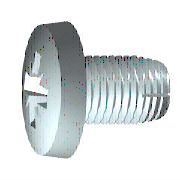
# Autodesk Inventor part: ANSI B18.6.5M - M3x0.5 x 16
Saved by Autodesk Inventor 2013 (Build 170138000, 138)
## iProperties
Created: 2012-02-10
Part Number: ANSI B18.6.5M - M3x0.5 x 16
Material: Steel, Mild
Description: Cross Recessed Pan Head Tapping Screw - Type D - Type IA - Metric
Document SubType Name: Modeling
Standard: ANSI B18.6.5M
Designer: Nico
Standard Revision: 2000
Standards Organization: ANSI
Language: en-US
Size Designation: M3x0.5 x 16
Categories: <MemberInstance><Categories><Category DisplayName="Fasteners" InternalName="e4da775c-781d-43d5-af7c-5136215cf5a6" Mnemonic="FSTN"><Category DisplayName="Bolts" InternalName="536e6df0-f778-49ac-b2f2-25c71d2aa0b2" Mnemonic="SCRW"><CategoryParameter DisplayName="Nominal Diameter" InternalName="8bbe3f8e-44cf-40a9-a251-3a6edc8168d6" Mnemonic="nomdia"/><CategoryParameter DisplayName="Nominal Length" InternalName="238ecbaf-3e6c-45dd-aa95-4068c8e0fd02" Mnemonic="nomlen"/><CategoryParameter DisplayName="Thread Series Designation" InternalName="87c5849c-b3a5-4c3e-9c9b-2feecef9be86" Mnemonic="thrserdsgn"/><CategoryParameter DisplayName="Thread Class" InternalName="ebc0d23b-2cc6-4d2a-b376-d52aae53bab6" Mnemonic="thrclss"/><CategoryParameter DisplayName="Thread Designation" InternalName="586d5e89-370a-4089-914f-0110033585c7" Mnemonic="thrdesign"/><CategoryParameter DisplayName="Thread Type" InternalName="b4bbb7bc-d6aa-4c9f-a9a9-4152b9f6fe49" Mnemonic="thrtype"/><CategoryParameter DisplayName="Threads per Unit" InternalName="bdc6e7d2-ffd0-4d9c-a173-16b95ebb912d" Mnemonic="thrperunit1"/><CategoryParameter DisplayName="Thread Pitch" InternalName="bb82302e-82d8-4176-8fc1-c5d7bb17d5ad" Mnemonic="pitch1"/><CategoryParameter DisplayName="Nominal Diameter Designation" InternalName="03caf894-eafd-4c09-a035-916ac084b87b" Mnemonic="nomdiadesig"/><Category DisplayName="Round Head" InternalName="df3578aa-538f-4805-96a8-2439eb0c3cf7" Mnemonic="RNDSCRW"><CategoryParameter DisplayName="Shank Diameter" InternalName="c22f1a48-b8d5-43ef-ac5e-546ba91c0bd6" Mnemonic="grpdia"/><CategoryParameter DisplayName="Grip Length" InternalName="2c6ace26-543b-4217-91c4-9cdf8c3ec6f1" Mnemonic="grplen"/><CategoryParameter DisplayName="Thread Length" InternalName="a1e5edc5-4ca7-4847-8786-65b14d35af16" Mnemonic="thrlen"/><CategoryParameter DisplayName="Head Diameter" InternalName="e71ee7a1-06fd-425c-ba3b-09769885677c" Mnemonic="headdia"/><CategoryParameter DisplayName="Head Height" InternalName="2d152238-84fe-49ae-94c3-3fee884c292b" Mnemonic="headh"/><CategoryParameter DisplayName="Property Class" InternalName="85496db6-1567-48ed-b0d4-aa1f03366005" Mnemonic="propclss"/><Category DisplayName="Self Tapping Screws" InternalName="33fb404f-0d7c-4133-a804-5105a5fcc9da" Mnemonic="RNDCNRGTPSCRW"/></Category></Category></Category><Category DisplayName="DataType" InternalName="23b78d0f-2648-40c6-8793-ca6db495c9e8" Mnemonic="DATATYPE"><CategoryParameter DisplayName="DisplayName" InternalName="05415f3d-3907-474b-a020-eb9d644f4cf3" Mnemonic="DISPLAYNAME"/><CategoryParameter DisplayName="InternalName" InternalName="cf1d0246-76d9-4b4a-8305-fa0409afb5c1" Mnemonic="INTERNALNAME"/><CategoryParameter DisplayName="Folder Name" InternalName="3f06958e-8713-4116-9be7-ed6184ecc97b" Mnemonic="FOLDERNAME"/><CategoryParameter DisplayName="Family Version" InternalName="914462f6-6e19-4b14-ba84-155b9680b1d0" Mnemonic="FAMILYREVISION"/><CategoryParameter DisplayName="ClipFormat" InternalName="bc51e27b-3422-4e78-93ef-cec197ddf230" Mnemonic="CLIPFORMAT"/><CategoryParameter DisplayName="IsMetric" InternalName="e2385c5b-1ea4-4823-96a8-8de651266ec3" Mnemonic="ISMETRIC"/><CategoryParameter DisplayName="Description" InternalName="13903e3d-64b1-4950-80da-f627842ea37f" Mnemonic="DESCRIPTION"/><CategoryParameter DisplayName="StdsOrg" InternalName="8f5914e1-4693-403f-8ab5-d37768198c9d" Mnemonic="STDSORG"/><CategoryParameter DisplayName="Standard" InternalName="0c0a119c-1e12-4c84-803f-101930972f5e" Mnemonic="STANDARD"/><CategoryParameter DisplayName="Manufacturer" InternalName="cd6c7a72-a28a-4e50-99a9-2c7f4e13e5ad" Mnemonic="MANUFACTURER"/><CategoryParameter DisplayName="Member Revision" InternalName="a65d44b9-392f-4f4f-857b-e4b3d54996fe" Mnemonic="MEMBERREVISION"/><CategoryParameter DisplayName="Standard Revision" InternalName="91d5a463-65c2-4fde-b823-3b7fea5e8e17" Mnemonic="STANDARDREVISION"/><CategoryParameter DisplayName="Revision Guid" InternalName="45a75005-10b1-4dfc-8d6d-dfe629f0b93c" Mnemonic="REVISIONGUID"/><CategoryParameter DisplayName="Designation" InternalName="2675968c-4ce5-49e0-a4f5-552d29089031" Mnemonic="DESIGNATION"/><CategoryParameter DisplayName="FileName" InternalName="8b46a4cc-9585-4fed-90c3-899f57e09a73" Mnemonic="FILENAME"/><CategoryParameter DisplayName="Default Row" InternalName="2af9ec52-faaa-4026-b378-f9fa4afca842" Mnemonic="DEFAULTROW"/><Category DisplayName="Part" InternalName="c0e0b642-3bcb-4cc8-9e80-f96d35c4afa4" Mnemonic="PART"><CategoryParameter DisplayName="Material" InternalName="818a152a-d3c3-49ca-80ee-df7d91421b8e" Mnemonic="MATERIAL"/><CategoryParameter DisplayName="Material Key" InternalName="5c9a8adb-dd2b-4535-b97f-0a94a95fe41f" Mnemonic="MATERIALKEY"/><CategoryParameter DisplayName="Part Number" InternalName="016b6077-bfbe-49bd-92c9-d8d59c39c941" Mnemonic="PARTNUMBER"/><CategoryParameter DisplayName="Stock Number" InternalName="4dba7c1c-e26c-444e-836c-b08b433409a8" Mnemonic="STOCKNUMBER"/></Category></Category><Category DisplayName="LegacyMap" InternalName="cd87c42b-3e48-431e-b5c0-1cbeb14dfe77" Mnemonic="LEGACYMAP"><CategoryParameter DisplayName="CatalogName" InternalName="d99d1e27-aa94-4de2-af4c-c348882a6f4f" Mnemonic="CATALOGNAME"/><CategoryParameter DisplayName="FamilyNumber" InternalName="e705e1f4-09cb-413e-91f9-551b4188271e" Mnemonic="FAMILYNUMBER"/><CategoryParameter DisplayName="MemberID" InternalName="8e5e0294-fc51-4c8f-b3d7-003dc5ed94f6" Mnemonic="MEMBERID"/><CategoryParameter DisplayName="unique CC member ID" InternalName="5193edd4-b2b0-4ab4-9d54-de900eee34e0" Mnemonic="CCCOOKIE"/><CategoryParameter DisplayName="unique DA member ID" InternalName="0918ad47-427f-4fed-ae26-24c81c58f590" Mnemonic="DACOOKIE"/><CategoryParameter DisplayName="Merge11 ID" InternalName="0ee8fb18-e2ed-4f39-96f6-1f4b5f50aa71" Mnemonic="MERGE11"/><CategoryParameter DisplayName="Split ID" InternalName="72b5c83c-be7f-45c4-ae51-9160ea6deb26" Mnemonic="SPLIT"/></Category></Categories><FamilyTemplate Id="si1048"><FamilyTemplateParameters><FamilyTemplateParameter ObjectType="kUserParameterObject" ValueType="xs:double" Id="1" ObjectReferenceKey="GUL"/><FamilyTemplateParameter ObjectType="kUserParameterObject" ValueType="xs:double" Id="2" ObjectReferenceKey="KOH"/><FamilyTemplateParameter ObjectType="kUserParameterObject" ValueType="xs:double" Id="3" ObjectReferenceKey="GD2"/><FamilyTemplateParameter ObjectType="kUserParameterObject" ValueType="xs:double" Id="4" ObjectReferenceKey="KOD"/><FamilyTemplateParameter ObjectType="kUserParameterObject" ValueType="xs:double" Id="5" ObjectReferenceKey="SBR"/><FamilyTemplateParameter ObjectType="kUserParameterObject" ValueType="xs:double" Id="6" ObjectReferenceKey="KR"/><FamilyTemplateParameter ObjectType="kUserParameterObject" ValueType="xs:double" Id="7" ObjectReferenceKey="GEL"/><FamilyTemplateParameter ObjectType="kUserParameterObject" ValueType="xs:double" Id="8" ObjectReferenceKey="THREADDIA"/><FamilyTemplateParameter ObjectType="kUserParameterObject" ValueType="xs:double" Id="9" ObjectReferenceKey="TOA"/><FamilyTemplateParameter ObjectType="kUserParameterObject" ValueType="xs:double" Id="10" ObjectReferenceKey="NLG"/><FamilyTemplateParameter ObjectType="kUserParameterObject" ValueType="xs:double" Id="11" ObjectReferenceKey="STI"/><FamilyTemplateParameter ObjectType="kUserParameterObject" ValueType="xs:double" Id="12" ObjectReferenceKey="TPU"/><FamilyTemplateParameter ObjectType="kUserParameterObject" ValueType="xs:double" Id="13" ObjectReferenceKey="PTC"/><FamilyTemplateParameter ObjectType="kUserParameterObject" ValueType="xs:double" Id="14" ObjectReferenceKey="SDM"/><FamilyTemplateParameter ObjectType="kUserParameterObject" ValueType="xs:double" Id="15" ObjectReferenceKey="NND"/><FamilyTemplateParameter ObjectType="kUserParameterObject" ValueType="xs:double" Id="16" ObjectReferenceKey="GAL"/><FamilyTemplateParameter ObjectType="kUserParameterObject" ValueType="xs:double" Id="17" ObjectReferenceKey="SPTZ"/><FamilyTemplateParameter ObjectType="kUserParameterObject" ValueType="xs:double" Id="18" ObjectReferenceKey="GD1"/><FamilyTemplateParameter ObjectType="kPropertyObject" ValueType="xs:string" Id="100" ObjectReferenceKey="{32853F0F-3444-11d1-9E93-0060B03C1CA6}" SubObjectId="52"/><FamilyTemplateParameter ObjectType="kPropertyObject" ValueType="xs:string" Id="105" ObjectReferenceKey="{32853F0F-3444-11d1-9E93-0060B03C1CA6}" SubObjectId="5"/><FamilyTemplateParameter ObjectType="kPartComponentDefinitionObject" ValueType="xs:string" Id="110" SubObjectId="Material"/><FamilyTemplateParameter ObjectType="kThreadFeatureObject" ValueType="xs:structure" Id="300" ObjectReferenceKey="1002000010000000aa0f0000000000008000000000000000" SubObjectId="ThreadInfo"><FamilyTemplateParameter ObjectType="" ValueType="xs:string" Id="301" SubObjectId="ThreadDesignation"/><FamilyTemplateParameter ObjectType="" ValueType="xs:string" Id="302" SubObjectId="ThreadClass"/><FamilyTemplateParameter ObjectType="" ValueType="xs:string" Id="303" SubObjectId="ThreadType"/></FamilyTemplateParameter></FamilyTemplateParameters></FamilyTemplate><CategoryParameterMap><ParamToTemplateMap><ParamToTemplate CategoryParameter="//CategoryParameter[@InternalName='05415f3d-3907-474b-a020-eb9d644f4cf3']" ConstantValue="Cross Recessed Pan Head Tapping Screw - Type D - Type IA - Metric"/><ParamToTemplate CategoryParameter="//CategoryParameter[@InternalName='cf1d0246-76d9-4b4a-8305-fa0409afb5c1']" ConstantValue="23d8e992-32c9-415c-94ef-986bdba1ac35"/><ParamToTemplate CategoryParameter="//CategoryParameter[@InternalName='3f06958e-8713-4116-9be7-ed6184ecc97b']" ConstantValue="ANSI B18.6.5M(23)"/><ParamToTemplate CategoryParameter="//CategoryParameter[@InternalName='914462f6-6e19-4b14-ba84-155b9680b1d0']" ConstantValue="10"/><ParamToTemplate CategoryParameter="//CategoryParameter[@InternalName='bc51e27b-3422-4e78-93ef-cec197ddf230']" ConstantValue="CF_INVENTOR.STDPARTS"/><ParamToTemplate CategoryParameter="//CategoryParameter[@InternalName='e2385c5b-1ea4-4823-96a8-8de651266ec3']" ConstantValue="true"/><ParamToTemplate CategoryParameter="//CategoryParameter[@InternalName='13903e3d-64b1-4950-80da-f627842ea37f']" ConstantValue="Cross Recessed Pan Head Tapping Screw - Type D - Type IA - Metric"/><ParamToTemplate CategoryParameter="//CategoryParameter[@InternalName='8f5914e1-4693-403f-8ab5-d37768198c9d']" ConstantValue="ANSI"/><ParamToTemplate CategoryParameter="//CategoryParameter[@InternalName='0c0a119c-1e12-4c84-803f-101930972f5e']" ConstantValue="ANSI B18.6.5M"/><ParamToTemplate CategoryParameter="//CategoryParameter[@InternalName='cd6c7a72-a28a-4e50-99a9-2c7f4e13e5ad']" TemplateParameter="104"/><ParamToTemplate CategoryParameter="//CategoryParameter[@InternalName='91d5a463-65c2-4fde-b823-3b7fea5e8e17']" ConstantValue="2000"/><ParamToTemplate CategoryParameter="//CategoryParameter[@InternalName='45a75005-10b1-4dfc-8d6d-dfe629f0b93c']" ConstantValue="689de755-fa26-4225-b770-7ed02537a583"/><ParamToTemplate CategoryParameter="//CategoryParameter[@InternalName='2af9ec52-faaa-4026-b378-f9fa4afca842']" ConstantValue="10"/><ParamToTemplate CategoryParameter="//CategoryParameter[@InternalName='d99d1e27-aa94-4de2-af4c-c348882a6f4f']" ConstantValue="ANSI"/><ParamToTemplate CategoryParameter="//CategoryParameter[@InternalName='e705e1f4-09cb-413e-91f9-551b4188271e']" ConstantValue="979"/><ParamToTemplate CategoryParameter="//CategoryParameter[@InternalName='8b46a4cc-9585-4fed-90c3-899f57e09a73']" ConstantValue="ANSI B18.6.5M - M3x0.5 x 16(39)"/><ParamToTemplate CategoryParameter="//CategoryParameter[@InternalName='a65d44b9-392f-4f4f-857b-e4b3d54996fe']" ConstantValue="f7747921-ac22-45e3-937a-a727b565ff1f"/><ParamToTemplate CategoryParameter="//CategoryParameter[@InternalName='c22f1a48-b8d5-43ef-ac5e-546ba91c0bd6']" ConstantValue="3"/><ParamToTemplate CategoryParameter="//CategoryParameter[@InternalName='2c6ace26-543b-4217-91c4-9cdf8c3ec6f1']" ConstantValue="0"/><ParamToTemplate CategoryParameter="//CategoryParameter[@InternalName='ebc0d23b-2cc6-4d2a-b376-d52aae53bab6']" ConstantValue="6g"/><ParamToTemplate CategoryParameter="//CategoryParameter[@InternalName='03caf894-eafd-4c09-a035-916ac084b87b']" ConstantValue="M3"/><ParamToTemplate CategoryParameter="//CategoryParameter[@InternalName='b4bbb7bc-d6aa-4c9f-a9a9-4152b9f6fe49']" ConstantValue="ISO Metric profile"/><ParamToTemplate CategoryParameter="//CategoryParameter[@InternalName='8e5e0294-fc51-4c8f-b3d7-003dc5ed94f6']" ConstantValue="180"/><ParamToTemplate CategoryParameter="//CategoryParameter[@InternalName='2675968c-4ce5-49e0-a4f5-552d29089031']" TemplateParameter="100"/><ParamToTemplate CategoryParameter="//CategoryParameter[@InternalName='a1e5edc5-4ca7-4847-8786-65b14d35af16']" TemplateParameter="7"/><ParamToTemplate CategoryParameter="//CategoryParameter[@InternalName='e71ee7a1-06fd-425c-ba3b-09769885677c']" TemplateParameter="4"/><ParamToTemplate CategoryParameter="//CategoryParameter[@InternalName='2d152238-84fe-49ae-94c3-3fee884c292b']" TemplateParameter="2"/><ParamToTemplate CategoryParameter="//CategoryParameter[@InternalName='818a152a-d3c3-49ca-80ee-df7d91421b8e']" TemplateParameter="110"/><ParamToTemplate CategoryParameter="//CategoryParameter[@InternalName='238ecbaf-3e6c-45dd-aa95-4068c8e0fd02']" TemplateParameter="10"/><ParamToTemplate CategoryParameter="//CategoryParameter[@InternalName='8bbe3f8e-44cf-40a9-a251-3a6edc8168d6']" TemplateParameter="15"/><ParamToTemplate CategoryParameter="//CategoryParameter[@InternalName='016b6077-bfbe-49bd-92c9-d8d59c39c941']" TemplateParameter="105"/><ParamToTemplate CategoryParameter="//CategoryParameter[@InternalName='bb82302e-82d8-4176-8fc1-c5d7bb17d5ad']" TemplateParameter="13"/><ParamToTemplate CategoryParameter="//CategoryParameter[@InternalName='586d5e89-370a-4089-914f-0110033585c7']" TemplateParameter="301"/><ParamToTemplate CategoryParameter="//CategoryParameter[@InternalName='bdc6e7d2-ffd0-4d9c-a173-16b95ebb912d']" TemplateParameter="12"/></ParamToTemplateMap></CategoryParameterMap></MemberInstance>
Density: 1 g/cm^3
IsCustomPart: 0
Author: Nico
Autodesk Inventor part; units mm, degrees
ref_plane "YZ Plane" through (0, 0, 0) normal (1, 0, 0) x (0, 1, 0)
sketch "Sketch1" plane through (0, 0, 0) normal (0, 0, 1) x (1, 0, 0)
  line L0 (25, 0) -> (25, 1.5)
  line L1 (25, 1.5) -> (0, 1.5)
  line L2 (3.9624, 5.08) -> (3.9624, 5.08)
  arc A0 (-1.6357, 2.6569) -> (-2.4, 0) centre (2.6, 0) ccw
  line L3 (-2.4, 0) -> (-2.4, 2.59)
  line L4 (-2.1961, 1.4133) -> (-0.7338, 0.6843)
  line L5 (-0.7338, 0.6843) -> (-0.37, 0)
  line L6 (-0.37, 0) -> (25, 0)
  line L7 (-6.3047, 0) -> (19.7175, 0) projected
  line L8 (0, -1.016) -> (0, 6.096) projected
  line L9 (-2.1961, 1.4133) -> (-2.4, 1.515) construction
  line L10 (-1.6357, 2.6569) -> (-2.4, 2.59)
  line L11 (-1.6357, 2.6569) -> (0, 2.8)
  line L12 (0, 2.8) -> (0, 1.5)
  dimension "d1" = 3
  dimension "d2" = 2.03
  dimension "d16" = 3.03
  dimension "d17" = 62
  dimension "d19" = 26.5
  dimension "d23" = 5.6
  dimension "d24" = 5
  dimension "d25" = 2.4
  dimension "d26" = 5
  dimension "d28" = 25
  constraints: 22 end point, 4 collinear, 4 point on circle, 3 point on line, 2 parallel, 1 centre point, 1 horizontal, 1 perpendicular, 1 tangent
  measures "d1" diameter of L1 L6
  measures "d2" distance from line of L5.end L3
  measures "d16" diameter of L9.end L6
  measures "d17" angle of L5 L6
  measures "d19" angle of L4 L6
  measures "d23" diameter of L11.end L6
  measures "d24" angle of L11 L6
  measures "d25" distance between parallel lines of L3 L12
  measures "d26" radius of A0
  measures "d28" distance between parallel lines of L0 L12
revolve "Body" add sketch "Sketch1" angle 360 about axis through (-0.37, 0, 0) along (1, 0, 0) contours L6 L8 L1 L0 | L8 L6 L5 L4 A0 L11
ref_plane "IDS_WORKPLANE{1}" through (-2.4, 0, 0) normal (1, 0, 0) x (0, 1, 0)
sketch "Sketch2" plane through (-2.4, 0, 0) normal (1, 0, 0) x (0, 1, 0)
  circle A0 centre (0, 0) radius 2.6569 projected
  line L0 (-4.5324, 0) -> (8.5962, 0) projected
  line L1 (0, -4.5324) -> (0, 8.5962) projected
  line L2 (0, 1.515) -> (0, 0) construction
  line L3 (0, 0) -> (1.515, 0) construction
  arc A1 (0.606, 0) -> (0, 0.606) centre (0, 0) ccw construction
  line L4 (0, 0) -> (6.7207, 6.7207) construction
  line L5 (0.365, 1.4704) -> (0.2198, 0.7249)
  line L6 (1.4704, 0.365) -> (0.7249, 0.2198)
  arc A2 (0.2198, 0.7249) -> (0.5495, 0.5495) centre (0.4114, 0.6876) ccw
  arc A3 (0.5495, 0.5495) -> (0.7249, 0.2198) centre (0.6876, 0.4114) ccw
  arc A4 (1.515, 0) -> (1.4704, 0.365) centre (0, 0) ccw
  arc A5 (0.365, 1.4704) -> (0, 1.515) centre (0, 0) ccw
  arc A6 (1.4704, 0.365) -> (0.365, 1.4704) centre (0, 0) ccw
  line L7 (0.365, -1.4704) -> (0.2198, -0.7249)
  line L8 (1.4704, -0.365) -> (0.7249, -0.2198)
  arc A7 (0.5495, -0.5495) -> (0.2198, -0.7249) centre (0.4114, -0.6876) ccw
  arc A8 (0.7249, -0.2198) -> (0.5495, -0.5495) centre (0.6876, -0.4114) ccw
  arc A9 (1.4704, -0.365) -> (1.515, 0) centre (0, 0) ccw
  arc A10 (0, -1.515) -> (0.365, -1.4704) centre (0, 0) ccw
  arc A11 (0.365, -1.4704) -> (1.4704, -0.365) centre (0, 0) ccw
  line L9 (-0.365, 1.4704) -> (-0.2198, 0.7249)
  line L10 (-1.4704, 0.365) -> (-0.7249, 0.2198)
  arc A12 (-0.5495, 0.5495) -> (-0.2198, 0.7249) centre (-0.4114, 0.6876) ccw
  arc A13 (-0.7249, 0.2198) -> (-0.5495, 0.5495) centre (-0.6876, 0.4114) ccw
  arc A14 (-1.4704, 0.365) -> (-1.515, 0) centre (0, 0) ccw
  arc A15 (0, 1.515) -> (-0.365, 1.4704) centre (0, 0) ccw
  arc A16 (-0.365, 1.4704) -> (-1.4704, 0.365) centre (0, 0) ccw
  arc A17 (-0.365, -1.4704) -> (0, -1.515) centre (0, 0) ccw
  arc A18 (-1.4704, -0.365) -> (-0.365, -1.4704) centre (0, 0) ccw
  arc A19 (-1.515, 0) -> (-1.4704, -0.365) centre (0, 0) ccw
  line L11 (-1.4704, -0.365) -> (-0.7249, -0.2198)
  line L12 (-0.365, -1.4704) -> (-0.2198, -0.7249)
  arc A20 (-0.2198, -0.7249) -> (-0.5495, -0.5495) centre (-0.4114, -0.6876) ccw
  arc A21 (-0.5495, -0.5495) -> (-0.7249, -0.2198) centre (-0.6876, -0.4114) ccw
  arc A22 (0.7575, 0) -> (0, 0.7575) centre (0, 0) ccw construction
  dimension "d4" = 45
  dimension "d5" = 1.212
  dimension "d6" = 3.03
  dimension "d7" = 0.365
  dimension "d20" = 1.515
  constraints: 46 point on circle, 25 symmetric about line, 22 centre point, 22 end point, 6 tangent, 4 coincident, 3 collinear, 3 point on line, 1 midpoint, 1 perpendicular, 22 other
  measures "d4" angle of L4 L3
  measures "d5" diameter of A1
  measures "d6" diameter of A6
  measures "d7" distance from line of L5.start L2
  measures "d20" diameter of A22
extrude "Slot" add sketch "Sketch2" along normal up to next draft 5 contours L6 A3 A2 L5 A6 | A11 L7 A7 A8 L8 | L9 A12 A13 L10 A16 | A18 L11 A21 A20 L12
revolve "Cut" cut sketch "Sketch1" angle 360 about axis through (-10, 0, 0) along (1, 0, 0) contours A0 L3 L10
sketch "Sketch4" plane through (-2.4, 0, 0) normal (1, 0, 0) x (0, 1, 0)
  circle A0 centre (0, 0) radius 2.6569 projected
  line L0 (-8.9998, 0) -> (8.9998, 0) projected
  line L1 (0, -8.9998) -> (0, 8.9998) projected
  line L2 (0, 0) -> (6.4284, 6.4284) construction
  circle A1 centre (0, 0) radius 0.1825 construction
  line L3 (0, 0) -> (6.4284, -6.4284) construction
  line L4 (0, 0) -> (-6.4284, 6.4284) construction
  line L5 (0, 0) -> (-6.4284, -6.4284) construction
  line L6 (1.0713, 1.0713) -> (0, 0.1825)
  line L7 (-1.0713, 1.0713) -> (-0.1825, 0)
  line L8 (-1.0713, -1.0713) -> (0, -0.1825)
  line L9 (1.0713, -1.0713) -> (0.1825, 0)
  line L10 (1.0713, 1.0713) -> (0.1825, 0)
  line L11 (-1.0713, 1.0713) -> (0, 0.1825)
  line L12 (-1.0713, -1.0713) -> (-0.1825, 0)
  line L13 (1.0713, -1.0713) -> (0, -0.1825)
  circle A2 centre (0, 0) radius 1.515 construction
  dimension "d11" = 0.365
  dimension "d14" = 45
  dimension "d31" = 1.0713
  constraints: 24 end point, 11 point on line, 7 point on circle, 3 symmetric about line, 2 centre point, 2 coincident, 2 perpendicular, 3 other
  measures "d11" diameter of A1
  measures "d14" angle of L2 L0
  measures "d31" distance from line of L0 L6.start
extrude "Star Cut" cut sketch "Sketch4" along normal blind 2.4 draft -30 contours L9 L13 L1 L0 | L0 L1 L6 L10 | L1 L0 L7 L11 | L8 L12 L0 L1
fillet "Fillet1" radius 0.146 5 edges at (-2.1961, 0, 1.4133) (-2.1961, -1.4133, 0) (-2.1961, 0, -1.4133) (-2.1961, 1.4036, -0.1652) (-2.1961, 1.4036, 0.1652)
thread "Thread" size "M3x0.5" class "6g" standard "ISO Metric profile" length 25
chamfer "Chamfer1" distance 0.34 distance2 0.5 1 edges at (25, -1.5, 0) measured on face at (25, -0.3888, 0.2119)
ref_plane "Work Plane3" through (12.5, 0, 0) normal (0, 0, -1) x (1, 0, 0)
equation "\"d5\" = 0.4 * SDM"
equation "\"d6\" = SDM"
equation "\"d7\" = 0.5 * SBR"
equation "\"d20\" = 0.5 * SDM"
equation "\"d11\" = 0.5 * SBR"
equation "\"d31\" = 0.353553 * SDM"
equation "\"d12\" = KOH"
equation "\"d1\" = NND"
equation "\"d2\" = STI"
equation "\"d16\" = SDM"
equation "\"d23\" = KOD"
equation "\"d25\" = KOH"
equation "\"d26\" = KR"
equation "\"d28\" = NLG"
equation "\"d22\" = 0.2 * SBR"
equation "\"d8\" = GEL"
equation "\"d29\" = -0.5 * GD2 + 0.5 * NND"
equation "\"d30\" = SPTZ"
equation "\"NND\" = 3"
equation "\"NLG\" = 25"
equation "\"GEL\" = 25"
equation "\"KOD\" = 5.6"
equation "\"KOH\" = 2.4"
equation "\"SDM\" = 3.03"
equation "\"STI\" = 2.03"
equation "\"SBR\" = 0.73"
equation "\"d3\" = -KOH"
equation "\"KR\" = 5"
equation "\"GD2\" = 2.32"
equation "\"SPTZ\" = 0.5"
equation "\"GUL\" = 0.61345 * PTC"
equation "\"THREADDIA\" = 3"
equation "\"TOA\" = 30deg"
equation "\"PTC\" = 0.5"
equation "\"GAL\" = 0.61345 * PTC"
equation "\"GD1\" = THREADDIA - 1.2269 * PTC"
body "Solid1"
